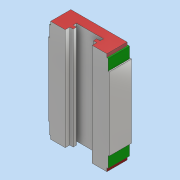
# Autodesk Inventor part: Wózek MGN12H
Saved by Autodesk Inventor 2018 (Build 220112000, 112)
## iProperties
Created: 2019-01-27
Part Number: Wózek MGN12H
Material: Ogólny
Document SubType Name: Modeling
Designer: Dawid
Density: 1 g/cm^3
Appearance: Aluminium — ciemne
Author: Dawid
Autodesk Inventor part; units mm, degrees
ref_plane "YZ Plane" through (0, 0, 0) normal (1, 0, 0) x (0, 1, 0)
ref_plane "XZ Plane" through (0, 0, 0) normal (0, 1, 0) x (-1, 0, 0)
ref_plane "XY Plane" through (0, 0, 0) normal (0, 0, 1) x (1, 0, 0)
sketch "Szkic1" plane through (0, 0, 0) normal (0, 0, 1) x (1, 0, 0)
  line L0 (6, 4) -> (-6, 4)
  line L1 (-6, 4) -> (-6, 2.5)
  line L2 (-6, 2.5) -> (-4.5, 2.5)
  line L3 (-4.5, 2.5) -> (-4.5, 1)
  line L4 (-4.5, 1) -> (-6, 1)
  line L5 (-6, 4) -> (-6, 2.5)
  line L6 (-6, 1) -> (-6, -1)
  line L7 (6, 4) -> (6, 2.5)
  line L8 (6, 2.5) -> (4.5, 2.5)
  line L9 (4.5, 2.5) -> (4.5, 1)
  line L10 (4.5, 1) -> (6, 1)
  line L11 (6, -1) -> (6, 1)
  line L12 (6, 2.5) -> (6, 4)
  line L13 (0, 9) -> (-13.5, 9)
  line L14 (0, 9) -> (13.5, 9)
  line L15 (-13.5, 9) -> (-13.5, -1)
  line L16 (13.5, -1) -> (13.5, 9)
  line L17 (-13.5, -1) -> (-6, -1)
  line L18 (6, -1) -> (13.5, -1)
  point P0 (0, 0)
  point P1 (0, 0)
  constraints: 38 end point, 9 perpendicular, 4 parallel, 1 horizontal, 1 vertical
extrude "Wyciągnięcie proste1" add sketch "Szkic1" along normal blind 32.4
sketch "Szkic2" plane through (-13.5, 9, 0) normal (0, 1, 0) x (1, 0, 0)
  line L0 (27, 0) -> (0, 0) projected
  line L1 (0, 0) -> (0, -32.4) projected
  line L2 (27, -32.4) -> (0, -32.4) projected
  line L3 (27, 0) -> (27, -32.4) projected
  line L4 (0, 0) -> (0, -32.4) projected
  line L5 (27, -32.4) -> (0, 0)
  line L6 (0, -32.4) -> (27, 0)
  line L7 (13.5, -6.2) -> (5, -6.2)
  line L8 (3.5, -7.7) -> (3.5, -24.7)
  line L9 (5, -26.2) -> (22, -26.2)
  line L10 (23.5, -24.7) -> (23.5, -7.7)
  line L11 (22, -6.2) -> (13.5, -6.2)
  circle A0 centre (3.5, -26.2) radius 1.5
  circle A1 centre (3.5, -6.2) radius 1.5
  circle A2 centre (23.5, -26.2) radius 1.5
  circle A3 centre (23.5, -6.2) radius 1.5
  point P0 (13.5, 0)
  dimension "d12" = 3
  dimension "d13" = 3
  dimension "d14" = 3
  dimension "d15" = 3
  constraints: 14 end point, 8 point on circle, 4 centre point, 3 perpendicular, 1 parallel
  measures "d12" diameter of A0
  measures "d13" diameter of A1
  measures "d14" diameter of A2
  measures "d15" diameter of A3
extrude "Wyciągnięcie proste2" cut sketch "Szkic2" against normal blind 3.5 contours A3 L6 | L6 A3 | A1 L5 | L5 A1 | A2 L5 | L5 A2 | A0 L6 | L6 A0
thread "Gwint1" size "M3x0.5" class "6H" standard "ANSI Metric M Profile" full length
thread "Gwint2" size "M3x0.5" class "6H" standard "ANSI Metric M Profile" full length
thread "Gwint3" size "M3x0.5" class "6H" standard "ANSI Metric M Profile" full length
thread "Gwint4" size "M3x0.5" class "6H" standard "ANSI Metric M Profile" full length
sketch "Szkic3" plane through (0, 0, 32.4) normal (0, 0, 1) x (1, 0, 0)
  line L0 (6, 4) -> (6, 2.5) projected
  line L1 (6, 2.5) -> (4.5, 2.5) projected
  line L2 (4.5, 2.5) -> (4.5, 1) projected
  line L3 (4.5, 1) -> (6, 1) projected
  line L4 (6, 1) -> (6, -1) projected
  line L5 (6, -1) -> (13.5, -1) projected
  line L6 (13.5, -1) -> (13.5, 9) projected
  line L7 (13.5, 9) -> (-13.5, 9) projected
  line L8 (-13.5, 9) -> (-13.5, -1) projected
  line L9 (-13.5, -1) -> (-6, -1) projected
  line L10 (-6, -1) -> (-6, 1) projected
  line L11 (-6, 1) -> (-4.5, 1) projected
  line L12 (-4.5, 1) -> (-4.5, 2.5) projected
  line L13 (-4.5, 2.5) -> (-6, 2.5) projected
  line L14 (-6, 2.5) -> (-6, 4) projected
  line L15 (-6, 4) -> (6, 4) projected
  line L16 (-13.5, -1) -> (-13, -1)
  line L17 (-13.5, -1) -> (-6, -1) projected
  line L18 (-13, -1) -> (-13, 8.5)
  line L19 (13.5, -1) -> (13, -1)
  line L20 (6, -1) -> (13.5, -1) projected
  line L21 (13, -1) -> (13, 8.5)
  line L22 (13, 8.5) -> (-13, 8.5)
  point P0 (0, 0)
  dimension "d26" = 0.5
  dimension "d27" = 0.5
  constraints: 10 end point, 2 perpendicular, 2 point on line
  measures "d26" distance of L8.end L16.end
  measures "d27" distance of L5.end L19.end
extrude "Wyciągnięcie proste3" add sketch "Szkic3" along normal blind 5 contours L15 L14 L13 L12 L11 L10 L9 L18 L22 L21 L5 L4 L3 L2 L1 L0
sketch "Szkic4" plane through (0, 0, 37.4) normal (0, 0, 1) x (1, 0, 0)
  line L0 (6, 4) -> (6, 2.5) projected
  line L1 (6, 2.5) -> (4.5, 2.5) projected
  line L2 (4.5, 2.5) -> (4.5, 1) projected
  line L3 (4.5, 1) -> (6, 1) projected
  line L4 (6, 1) -> (6, -1) projected
  line L5 (6, -1) -> (13, -1) projected
  line L6 (13, -1) -> (13, 8.5) projected
  line L7 (13, 8.5) -> (-13, 8.5) projected
  line L8 (-13, 8.5) -> (-13, -1) projected
  line L9 (-13, -1) -> (-6, -1) projected
  line L10 (-6, -1) -> (-6, 1) projected
  line L11 (-6, 1) -> (-4.5, 1) projected
  line L12 (-4.5, 1) -> (-4.5, 2.5) projected
  line L13 (-4.5, 2.5) -> (-6, 2.5) projected
  line L14 (-6, 2.5) -> (-6, 4) projected
  line L15 (-6, 4) -> (6, 4) projected
  line L16 (-13, -1) -> (-12.5, -1)
  line L17 (-13.5, -1) -> (-6, -1) projected
  line L18 (-12.5, -1) -> (-12.5, 8)
  line L19 (13, -1) -> (12.5, -1)
  line L20 (6, -1) -> (13.5, -1) projected
  line L21 (12.5, -1) -> (12.5, 8)
  line L22 (12.5, 8) -> (-12.5, 8)
  point P0 (0, 0)
  constraints: 10 end point, 3 perpendicular, 2 point on line
extrude "Wyciągnięcie proste4" add sketch "Szkic4" along normal blind 1.5 contours L15 L14 L13 L12 L11 L10 L9 L18 L22 L21 L5 L4 L3 L2 L1 L0
sketch "Szkic5" plane through (0, 0, 0) normal (0, 0, -1) x (-1, 0, 0)
  line L0 (-6, -1) -> (-13, -1)
  line L1 (-6, 4) -> (-6, 2.5)
  line L2 (6, 4) -> (-6, 4)
  line L3 (6, 2.5) -> (6, 4)
  line L4 (4.5, 2.5) -> (6, 2.5)
  line L5 (4.5, 1) -> (4.5, 2.5)
  line L6 (6, 1) -> (4.5, 1)
  line L7 (6, -1) -> (6, 1)
  line L8 (-6, -1) -> (-13, -1)
  line L9 (-6, 1) -> (-6, -1)
  line L10 (-4.5, 1) -> (-6, 1)
  line L11 (-4.5, 2.5) -> (-4.5, 1)
  line L12 (-6, 2.5) -> (-4.5, 2.5)
  line L13 (13.5, -1) -> (6, -1) projected
  line L14 (6, -1) -> (13, -1)
  line L15 (-6, 4) -> (-6, 2.5) projected
  line L16 (6, 4) -> (-6, 4) projected
  line L17 (6, 2.5) -> (6, 4) projected
  line L18 (4.5, 2.5) -> (6, 2.5) projected
  line L19 (4.5, 1) -> (4.5, 2.5) projected
  line L20 (6, 1) -> (4.5, 1) projected
  line L21 (6, -1) -> (6, 1) projected
  line L22 (13.5, -1) -> (6, -1) projected
  line L23 (13.5, 9) -> (13.5, -1) projected
  line L24 (-13.5, 9) -> (13.5, 9) projected
  line L25 (-13.5, -1) -> (-13.5, 9) projected
  line L26 (-6, -1) -> (-13.5, -1) projected
  line L27 (-6, 1) -> (-6, -1) projected
  line L28 (-4.5, 1) -> (-6, 1) projected
  line L29 (-4.5, 2.5) -> (-4.5, 1) projected
  line L30 (-6, 2.5) -> (-4.5, 2.5) projected
  line L31 (-13.5, -1) -> (-13.5, 9) projected
  line L32 (-13.5, 9) -> (-13, 9)
  line L33 (-13, -1) -> (-13, 8.5) projected
  line L34 (-13, 9) -> (-13, -1)
  line L35 (13.5, 9) -> (13, 9)
  line L36 (-13.5, 9) -> (13.5, 9) projected
  line L37 (13, 9) -> (13, -1)
  line L38 (-13, 9) -> (-13, 8.5)
  line L39 (13, 8.5) -> (-13, 8.5) projected
  line L40 (-13, 8.5) -> (13, 8.5)
  point P0 (0, 0)
  dimension "d45" = 0.5
  dimension "d46" = 0.5
  dimension "d47" = 0.5
  dimension "d49" = 26
  constraints: 40 end point, 2 collinear, 2 point on line, 1 perpendicular
  measures "d45" distance of L24.start L32.end
  measures "d46" distance of L23.start L35.end
  measures "d47" distance of L32.end L33.end
  measures "d49" distance of L33.end L39.start
extrude "Wyciągnięcie proste5" add sketch "Szkic5" along normal blind 5 contours L0 L33 L39 L37 L13 L7 L6 L5 L4 L3 L2 L1 L12 L11 L10 L9
sketch "Szkic7" plane through (0, 0, -5) normal (0, 0, -1) x (-1, 0, 0)
  line L0 (-13, -1) -> (-6, -1)
  line L1 (-6, -1) -> (-6, 1)
  line L2 (-6, 1) -> (-4.5, 1)
  line L3 (-4.5, 1) -> (-4.5, 2.5)
  line L4 (-4.5, 2.5) -> (-6, 2.5)
  line L5 (-6, 2.5) -> (-6, 4)
  line L6 (-6, 4) -> (6, 4)
  line L7 (6, 4) -> (6, 2.5)
  line L8 (6, 2.5) -> (4.5, 2.5)
  line L9 (4.5, 2.5) -> (4.5, 1)
  line L10 (4.5, 1) -> (6, 1)
  line L11 (6, 1) -> (6, -1)
  line L12 (6, -1) -> (13, -1)
  line L13 (-6, -1) -> (-12.5, -1)
  line L14 (-13, -1) -> (-12.5, -1)
  line L15 (-12.5, -1) -> (-12.5, 8)
  line L16 (13, -1) -> (12.5, -1)
  line L17 (6, -1) -> (13, -1)
  line L18 (12.5, -1) -> (12.5, 8)
  line L19 (12.5, 8) -> (12.5, -1)
  line L20 (-12.5, -1) -> (-12.5, 8)
  line L21 (12.5, 8) -> (-12.5, 8)
  point P0 (0, 0)
  dimension "d53" = 25
  dimension "d54" = 9
  dimension "d55" = 9
  constraints: 44 end point, 1 point on line
  measures "d53" distance of L18.end L15.end
  measures "d54" distance of L13.end L15.end
  measures "d55" distance of L18.end L16.end
extrude "Wyciągnięcie proste6" add sketch "Szkic7" along normal blind 1.5
sketch "Szkic8" plane through (-13.5, 9, 0) normal (0, 1, 0) x (1, 0, 0)
  circle A0 centre (23.5, -6.2) radius 1.5 projected
  circle A1 centre (23.5, -26.2) radius 1.5 projected
  circle A2 centre (3.5, -6.2) radius 1.5 projected
  circle A3 centre (3.5, -26.2) radius 1.5 projected
  line L0 (27, 0) -> (0, 0) projected
  line L1 (0, 0) -> (0, -32.4) projected
  line L2 (27, -32.4) -> (0, -32.4) projected
  line L3 (27, 0) -> (27, -32.4) projected
  line L4 (27, 0) -> (27, -32.4) projected
  line L5 (27, 0) -> (20, 0)
  line L6 (20, 0) -> (20, -32.4)
  line L7 (0, -32.4) -> (7, -32.4)
  line L8 (27, -32.4) -> (0, -32.4) projected
  line L9 (7, -32.4) -> (7, 0)
  point P0 (13.5, 0)
  dimension "d58" = 7
  dimension "d59" = 7
  constraints: 8 end point, 4 point on line, 2 perpendicular
  measures "d58" distance of L0.start L5.end
  measures "d59" distance of L1.end L7.end
extrude "Wyciągnięcie proste7" cut sketch "Szkic8" against normal blind 0.25 contours L6 L2 L9 L0
